Respeaker Zero Case (Autodesk Fusion 360 design; units mm, degrees)
Autodesk Fusion 360 part; units mm, degrees
sketch "Base Bottom" plane through (0, 0, 0) normal (0, 1, 0) x (1, 0, 0)
  line L0 (0, 0) -> (66.3, 0)
  line L1 (66.3, 0) -> (66.3, -31)
  line L2 (66.3, -31) -> (0, -31)
  line L3 (0, -31) -> (0, 0)
  line L4 (-2, -33) -> (68.3, -33)
  line L5 (68.3, -33) -> (68.3, 2)
  line L6 (68.3, 2) -> (-2, 2)
  line L7 (-2, 2) -> (-2, -33)
  line L8 (60, -31) -> (50, -31)
  line L9 (50, -31) -> (50, -33)
  line L10 (50, -33) -> (60, -33)
  line L11 (60, -33) -> (60, -31)
  line L12 (7.15, -7.5) -> (59.15, -7.5)
  line L13 (59.15, -7.5) -> (59.15, 0)
  line L14 (59.15, 0) -> (7.15, 0)
  line L15 (7.15, 0) -> (7.15, -7.5)
  line L16 (-2, -20.5) -> (0, -20.5)
  line L17 (0, -20.5) -> (0, -6.5)
  line L18 (0, -6.5) -> (-2, -6.5)
  line L19 (-2, -6.5) -> (-2, -20.5)
  dimension "d1" = 31
  dimension "d2" = 66.3
  dimension "d3" = 2
  dimension "d4" = 2
  dimension "d5" = 2
  dimension "d6" = 2
  dimension "d9" = 10
  dimension "d12" = 52
  dimension "d13" = 7.5
  dimension "d14" = 7.15
  dimension "d38" = 14
  dimension "d39" = 10.5
  dimension "d40" = 50
  constraint horizontal L0
  constraint vertical L1
  constraint horizontal L2
  constraint vertical L3
  constraint coincident L0.start L3.end
  constraint horizontal L4
  constraint vertical L5
  constraint horizontal L6
  constraint vertical L7
  constraint horizontal L8
  constraint vertical L9
  constraint horizontal L10
  constraint vertical L11
  constraint coincident L4 L9.end
  constraint coincident L2 L8.start
  constraint horizontal L12
  constraint vertical L13
  constraint horizontal L14
  constraint vertical L15
  constraint horizontal L16
  constraint vertical L17
  constraint horizontal L18
  constraint vertical L19
  constraint collinear L3 L17
  constraint collinear L7 L19
  constraint collinear L0 L14
  measures "d1" distance of L0.start L2.end
  measures "d2" distance of L0.start L0.end
  measures "d3" distance of L2 L4
  measures "d4" distance of L1 L5
  measures "d5" distance of L0 L6
  measures "d6" distance of L3 L7
  measures "d9" distance of L8.start L8.end
  measures "d12" distance of L12.start L12.end
  measures "d13" distance of L12.start L14.end
  measures "d14" horizontal distance of L0.start L14.end
  measures "d38" distance of L16.start L18.end
  measures "d39" distance of L2.end L16.end
  measures "d40" distance of L2.end L8.end
  measures "d53" distance of L0.end
  measures "d63" distance of L0.end
  measures "d64" distance of L0.end
extrude "Extrude1" add sketch "Base Bottom" along normal blind 1 makes body 1
extrude "Extrude2" add sketch "Base Bottom" along normal blind 3.5 contours L0 L1 L2 L3 L8 L12 L13 L15 L17 bodies 1
extrude "Extrude3" add sketch "Base Bottom" along normal blind 14 contours L0 L1 L2 L3 L4 L5 L6 L7 L11 L14 L18 | L3 L7 L16 L17 L18 L19 | L2 L3 L4 L7 L9 L16 | L2 L4 L8 L9 L10 L11 bodies 1
sketch "Base Back USB" plane through (0, 0, 33) normal (0, 0, 1) x (-1, 0, 0)
  line L0 (2, 0) -> (-68.3, 0)
  line L1 (-68.3, 0) -> (-68.3, -14)
  line L2 (-68.3, -14) -> (2, -14)
  line L3 (2, -14) -> (2, 0)
  line L4 (-50, -3.5) -> (-60, -3.5)
  line L5 (-60, -3.5) -> (-60, -9.5)
  line L6 (-60, -9.5) -> (-50, -9.5)
  line L7 (-50, -9.5) -> (-50, -3.5)
  line L8 (2, 0) -> (-68.3, 0)
  dimension "d22" = 10
  dimension "d23" = 6
  dimension "d27" = 3.5
  dimension "d41" = 52
  constraint horizontal L4
  constraint vertical L5
  constraint horizontal L6
  constraint vertical L7
  measures "d22" distance of L4.start L4.end
  measures "d23" distance of L4.start L6.end
  measures "d27" distance of L4.start L8
  measures "d41" distance of L3 L6.end
ref_plane "WorkPlane1" through (33.15, 3.5, 15.5) normal (0, 1, 0) x (0, 0, 1)
extrude "Extrude4" cut sketch "Base Back USB" against normal blind 13 contours L4 L5 L6 L7 bodies 1
sketch "Base Side SD" plane through (-2, 0, 0) normal (-1, 0, 0) x (0, -1, 0)
  line L0 (0, -2) -> (0, 33)
  line L1 (0, 33) -> (-14, 33)
  line L2 (-14, 33) -> (-14, -2)
  line L3 (-14, -2) -> (0, -2)
  line L4 (-8, 20.5) -> (-4, 20.5)
  line L5 (-4, 20.5) -> (-4, 6.5)
  line L6 (-4, 6.5) -> (-8, 6.5)
  line L7 (-8, 6.5) -> (-8, 20.5)
  line L8 (0, 6.5) -> (0, 20.5)
  point P0 (0, 33)
  dimension "d42" = 14
  dimension "d43" = 4
  dimension "d44" = 4
  dimension "d127" = 8.5
  constraint horizontal L4
  constraint vertical L5
  constraint horizontal L6
  constraint vertical L7
  measures "d42" distance of L4.start L6.end
  measures "d43" distance of L4.start L4.end
  measures "d44" distance of L5 L8
  measures "d127" distance of L3 L6
extrude "Extrude6" cut sketch "Base Side SD" against normal blind 4 contours L4 L5 L6 L7 bodies 1
sketch "Base Front Mic" plane through (0, 0, -2) normal (0, 0, -1) x (1, 0, 0)
  line L0 (68.3, 0) -> (-2, 0)
  line L1 (-2, 0) -> (-2, -14)
  line L2 (-2, -14) -> (68.3, -14)
  line L3 (68.3, -14) -> (68.3, 0)
  line L4 (64.8, -10.35) -> (59.8, -10.35)
  line L5 (59.8, -10.35) -> (59.8, -14)
  line L6 (59.8, -14) -> (64.8, -14)
  line L7 (64.8, -14) -> (64.8, -10.35)
  line L8 (68.3, 0) -> (-2, 0)
  line L9 (1.5, -10.35) -> (6.5, -10.35)
  line L10 (6.5, -10.35) -> (6.5, -14)
  line L11 (6.5, -14) -> (1.5, -14)
  line L12 (1.5, -14) -> (1.5, -10.35)
  dimension "d48" = 3.5
  dimension "d49" = 10.35
  dimension "d50" = 5
  dimension "d51" = 3.5
  dimension "d52" = 10.35
  dimension "d53" = 5
  constraint horizontal L4
  constraint vertical L5
  constraint horizontal L6
  constraint vertical L7
  constraint coincident L2 L6.end
  constraint horizontal L9
  constraint vertical L10
  constraint horizontal L11
  constraint vertical L12
  constraint coincident L2 L11.end
  measures "d48" distance of L3 L7
  measures "d49" distance of L4 L8
  measures "d50" distance of L4.start L4.end
  measures "d51" distance of L1 L12
  measures "d52" distance of L8 L9
  measures "d53" distance of L10.end L11.end
extrude "Extrude7" cut sketch "Base Front Mic" against normal blind 4 contours L2 L4 L5 L6 L7 | L2 L9 L10 L11 L12 bodies 1
sketch "Base Side Serial" plane through (68.3, 0, 0) normal (1, 0, 0) x (0, 1, 0)
  line L0 (0, 33) -> (0, -2)
  line L1 (0, -2) -> (14, -2)
  line L2 (14, -2) -> (14, 33)
  line L3 (14, 33) -> (0, 33)
  line L4 (4, 24.5) -> (8, 24.5)
  line L5 (8, 24.5) -> (8, 6.5)
  line L6 (8, 6.5) -> (4, 6.5)
  line L7 (4, 6.5) -> (4, 24.5)
  dimension "d113" = 4
  dimension "d114" = 18
  dimension "d115" = 4
  dimension "d128" = 8.5
  constraint horizontal L4
  constraint vertical L5
  constraint horizontal L6
  constraint vertical L7
  measures "d113" distance of L4.start L4.end
  measures "d114" distance of L4.end L5.end
  measures "d115" distance of L0 L7
  measures "d128" distance of L1 L6
extrude "Extrude14" cut sketch "Base Side Serial" against normal blind 10 contours L4 L5 L6 L7 bodies 1
sketch "Cap" plane through (0, 0, 0) normal (0, 1, 0) x (1, 0, 0)
  line L0 (0, 0) -> (66.3, 0)
  line L1 (66.3, 0) -> (66.3, -31)
  line L2 (66.3, -31) -> (0, -31)
  line L3 (0, -31) -> (0, 0)
  line L4 (68.3, -33) -> (-2, -33)
  line L5 (-2, -33) -> (-2, 2)
  line L6 (-2, 2) -> (68.3, 2)
  line L7 (68.3, 2) -> (68.3, -33)
  line L8 (64.3, -29) -> (2, -29)
  line L9 (2, -29) -> (2, -2)
  line L10 (2, -2) -> (64.3, -2)
  line L11 (64.3, -2) -> (64.3, -29)
  line L12 (64.8, -10.5) -> (61.3, -10.5)
  line L13 (61.3, -10.5) -> (61.3, 0)
  line L14 (61.3, 0) -> (64.8, 0)
  line L15 (64.8, 0) -> (64.8, -10.5)
  line L16 (64.8, -10.5) -> (60.3, -10.5)
  line L17 (60.3, -10.5) -> (60.3, -11.5)
  line L18 (60.3, -11.5) -> (64.8, -11.5)
  line L19 (64.8, -11.5) -> (64.8, -10.5)
  line L20 (5, -10.5) -> (1.5, -10.5)
  line L21 (1.5, -10.5) -> (1.5, 0)
  line L22 (1.5, 0) -> (5, 0)
  line L23 (5, 0) -> (5, -10.5)
  line L24 (1.5, -10.5) -> (6, -10.5)
  line L25 (6, -10.5) -> (6, -11.5)
  line L26 (6, -11.5) -> (1.5, -11.5)
  line L27 (1.5, -11.5) -> (1.5, -10.5)
  line L28 (6, -10.5) -> (5, -10.5)
  line L29 (5, -10.5) -> (5, 0)
  line L30 (5, 0) -> (6.5, 0)
  line L31 (64.8, -10.5) -> (66.3, -10.5)
  line L32 (66.3, -10.5) -> (66.3, -11.5)
  line L33 (66.3, -11.5) -> (64.8, -11.5)
  line L34 (64.8, -11.5) -> (64.8, -10.5)
  line L35 (1.5, -11.5) -> (0, -11.5)
  line L36 (0, -11.5) -> (0, -10.5)
  line L37 (0, -10.5) -> (1.5, -10.5)
  line L38 (1.5, -10.5) -> (1.5, -11.5)
  circle A0 centre (49, -12.4) radius 3.3
  line L39 (66.3, -11.5) -> (64.3, -11.5)
  line L40 (64.3, -11.5) -> (64.3, -21)
  line L41 (64.3, -21) -> (66.3, -21)
  line L42 (66.3, -21) -> (66.3, -11.5)
  line L43 (1.5, 0) -> (6.5, 0)
  line L44 (6.5, 0) -> (6.5, 2)
  line L45 (6.5, 2) -> (1.5, 2)
  line L46 (1.5, 2) -> (1.5, 0)
  line L47 (59.8, 0) -> (64.8, 0)
  line L48 (64.8, 0) -> (64.8, 2)
  line L49 (64.8, 2) -> (59.8, 2)
  line L50 (59.8, 2) -> (59.8, 0)
  line L51 (5, -10.5) -> (6, -10.5)
  line L52 (6, -10.5) -> (6, -7.3)
  line L53 (6, -7.3) -> (5, -7.3)
  line L54 (5, -7.3) -> (5, -10.5)
  line L55 (5, -7.3) -> (6.5199, 0.1987)
  line L56 (6.5199, 0.1987) -> (7.5, 0)
  line L57 (7.5, 0) -> (5.9801, -7.4987)
  line L58 (5.9801, -7.4987) -> (5, -7.3)
  line L59 (61.3, -10.5) -> (60.3, -10.5)
  line L60 (60.3, -10.5) -> (60.3, -7.3)
  line L61 (60.3, -7.3) -> (61.3, -7.3)
  line L62 (61.3, -7.3) -> (61.3, -10.5)
  line L63 (61.3, -7.3) -> (59.7801, 0.1987)
  line L64 (59.7801, 0.1987) -> (58.8, 0)
  line L65 (58.8, 0) -> (60.3199, -7.4987)
  line L66 (60.3199, -7.4987) -> (61.3, -7.3)
  dimension "d56" = 66.3
  dimension "d57" = 31
  dimension "d58" = 2
  dimension "d59" = 2
  dimension "d60" = 2
  dimension "d61" = 2
  dimension "d62" = 2
  dimension "d63" = 2
  dimension "d64" = 2
  dimension "d65" = 2
  dimension "d72" = 3.5
  dimension "d73" = 3.5
  dimension "d74" = 10.5
  dimension "d75" = 4.5
  dimension "d76" = 1
  dimension "d78" = 3.5
  dimension "d79" = 3.5
  dimension "d80" = 10.5
  dimension "d81" = 4.5
  dimension "d82" = 1
  dimension "d103" = 6.6
  dimension "d105" = 14.4
  dimension "d108" = 19.3
  dimension "d109" = 9.5
  dimension "d129" = 3.5
  dimension "d130" = 5
  dimension "d131" = 5
  dimension "d132" = 3.5
  dimension "d137" = 1
  dimension "d138" = 3.2
  dimension "d139" = 1
  dimension "d140" = 6
  dimension "d141" = 1
  dimension "d142" = 3.2
  dimension "d143" = 1
  dimension "d144" = 6
  constraint horizontal L0
  constraint vertical L1
  constraint horizontal L2
  constraint vertical L3
  constraint coincident L0.start L3.end
  constraint horizontal L4
  constraint vertical L5
  constraint horizontal L6
  constraint vertical L7
  constraint horizontal L8
  constraint vertical L9
  constraint horizontal L10
  constraint vertical L11
  constraint horizontal L12
  constraint vertical L13
  constraint horizontal L14
  constraint vertical L15
  constraint coincident L0 L13.end
  constraint horizontal L16
  constraint vertical L17
  constraint horizontal L18
  constraint vertical L19
  constraint horizontal L20
  constraint vertical L21
  constraint horizontal L22
  constraint vertical L23
  constraint coincident L0 L21.end
  constraint horizontal L24
  constraint vertical L25
  constraint horizontal L26
  constraint vertical L27
  constraint horizontal L28
  constraint vertical L29
  constraint horizontal L30
  constraint horizontal L31
  constraint vertical L32
  constraint horizontal L33
  constraint vertical L34
  constraint coincident L1 L32.end
  constraint horizontal L35
  constraint vertical L36
  constraint horizontal L37
  constraint vertical L38
  constraint coincident L3 L36.end
  constraint horizontal L39
  constraint vertical L40
  constraint horizontal L41
  constraint vertical L42
  constraint collinear L11 L40
  constraint horizontal L43
  constraint vertical L44
  constraint horizontal L45
  constraint vertical L46
  constraint collinear L0 L43
  constraint collinear L6 L45
  constraint horizontal L47
  constraint vertical L48
  constraint horizontal L49
  constraint vertical L50
  constraint collinear L0 L47
  constraint collinear L6 L49
  constraint horizontal L51
  constraint vertical L52
  constraint horizontal L53
  constraint vertical L54
  constraint perpendicular L55 L56
  constraint parallel L55 L57
  constraint parallel L56 L58
  constraint coincident L0 L56.end
  constraint horizontal L59
  constraint vertical L60
  constraint horizontal L61
  constraint vertical L62
  constraint perpendicular L63 L64
  constraint parallel L63 L65
  constraint parallel L64 L66
  constraint coincident L0 L64.end
  measures "d56" distance of L1.end L2.end
  measures "d57" distance of L0.end L1.end
  measures "d58" distance of L2 L4
  measures "d59" distance of L3 L5
  measures "d60" distance of L0 L6
  measures "d61" distance of L1 L7
  measures "d62" distance of L2 L8
  measures "d63" distance of L1 L11
  measures "d64" distance of L0 L10
  measures "d65" distance of L3 L9
  measures "d72" distance of L7 L15
  measures "d73" distance of L12.start L12.end
  measures "d74" distance of L12.end L13.end
  measures "d75" distance of L12.start L16.end
  measures "d76" distance of L12.start L18.end
  measures "d78" distance of L5 L21
  measures "d79" distance of L20.start L20.end
  measures "d80" distance of L20.start L22.end
  measures "d81" distance of L20.end L24.end
  measures "d82" distance of L20.end L26.end
  measures "d103" diameter of A0
  measures "d105" distance of L6 A0.centre
  measures "d108" distance of L7 A0.centre
  measures "d109" distance of L32.end L41.end
  measures "d129" distance of L5 L46
  measures "d130" distance of L44.end L45.end
  measures "d131" distance of L48.end L49.end
  measures "d132" distance of L7 L48
  measures "d137" distance of L20.start L24.end
  measures "d138" distance of L20.start L53.end
  measures "d139" distance of L53.end L57.end
  measures "d140" distance of L21 L56.end
  measures "d141" distance of L12.end L16.end
  measures "d142" distance of L16.end L60.end
  measures "d143" distance of L61.end L65.end
  measures "d144" distance of L15 L64.end
extrude "Extrude8" add sketch "Cap" along normal blind 2 separate body contours L0 L1 L2 L3 L4 L5 L6 L7 L32 L36 L42 L46 L48 | L0 L3 L21 L37 | L0 L6 L22 L30 L43 L44 L45 L46 L55 | L0 L9 L10 L20 L21 L22 L23 L24 L29 L43 | L3 L27 L35 L36 L37 L38 | L0 L10 L23 L29 L30 L43 L55 | L9 L20 L24 L26 L27 L38 | L1 L2 L3 L8 L9 L11 L26 L35 L41 | L0 L30 L43 L44 L55 | L0 L10 L30 L43 L55 L57 | L9 L10 L20 L23 L24 L29 L54 | L10 L23 L29 L55 | L9 L20 L24 L25 L26 L28 L51 | L0 L6 L44 L50 L55 L56 L63 L64 | L0 L44 L55 L56 | L10 L52 L53 L55 L57 | L23 L24 L28 L29 L51 L52 L54 L57 L58 | L52 L53 L57 L58 | L8 L9 L10 L11 L17 L18 L25 L26 L40 L52 L57 L60 L65 | L0 L6 L14 L47 L48 L49 L50 L63 | L0 L10 L57 L65 | L0 L47 L50 L63 | L0 L50 L63 L64 | L1 L11 L18 L33 L39 L40 L41 L42 | L0 L10 L47 L63 L65 | L10 L60 L61 L63 L65 | L0 L10 L11 L12 L13 L14 L15 L16 L47 | L0 L1 L15 L31 | L0 L10 L13 L47 L63 | L1 L19 L31 L32 L33 L34 L39 | L10 L13 L63 | L13 L16 L59 L60 L62 L65 L66 | L60 L61 L65 L66 | L11 L12 L16 L18 L19 L34 L39 | L11 L12 L16 L17 L18 L59 | L10 L11 L12 L13 L16 L62 | A0 makes body 2
extrude "Extrude9" add sketch "Cap" along normal blind 4 contours L0 L3 L21 L37 | L0 L9 L10 L20 L21 L22 L23 L24 L29 L43 | L3 L27 L35 L36 L37 L38 | L0 L10 L23 L29 L30 L43 L55 | L9 L20 L24 L26 L27 L38 | L1 L2 L3 L8 L9 L11 L26 L35 L41 | L0 L10 L30 L43 L55 L57 | L0 L10 L57 L65 | L1 L11 L18 L33 L39 L40 L41 L42 | L0 L10 L47 L63 L65 | L0 L10 L11 L12 L13 L14 L15 L16 L47 | L0 L1 L15 L31 | L0 L10 L13 L47 L63 | L1 L19 L31 L32 L33 L34 L39 | L11 L12 L16 L18 L19 L34 L39 bodies 2
extrude "Extrude10" cut sketch "Cap" along normal blind 2 from surface at 2 contours L0 L9 L10 L20 L21 L22 L23 L24 L29 L43 | L0 L10 L23 L29 L30 L43 L55 | L0 L10 L47 L63 L65 | L0 L10 L11 L12 L13 L14 L15 L16 L47 | L0 L10 L13 L47 L63 bodies 2
extrude "Extrude11" add sketch "Cap" along normal blind 3.6 from surface at 2 contours L0 L3 L21 L37 | L3 L27 L35 L36 L37 L38 | L9 L20 L24 L26 L27 L38 | L0 L10 L30 L43 L55 L57 | L9 L20 L24 L25 L26 L28 L51 | L10 L52 L53 L55 L57 | L23 L24 L28 L29 L51 L52 L54 L57 L58 | L52 L53 L57 L58 | L0 L10 L47 L63 L65 | L10 L60 L61 L63 L65 | L0 L1 L15 L31 | L1 L19 L31 L32 L33 L34 L39 | L13 L16 L59 L60 L62 L65 L66 | L60 L61 L65 L66 | L11 L12 L16 L18 L19 L34 L39 | L11 L12 L16 L17 L18 L59 bodies 2
extrude "Extrude12" cut sketch "Cap" along normal blind 6 contours A0 bodies 2
extrude "Extrude13" cut sketch "Cap" along normal blind 3 from surface at 2 contours L1 L11 L18 L33 L39 L40 L41 L42 bodies 2
fillet "Fillet1" radius 4.5 2 edges at (63.05, 2, 10.5) (3.25, 2, 10.5) on bodies 2
copy_body "Body->Comp1" bodies 1 removing the originals makes body 3 in component "Base"
copy_body "Body->Comp2" bodies 2 removing the originals makes body 4 in component "Cap"
chamfer "Chamfer1" distance 2 angle 45 6 edges at (62.3, 10.35, -2) (64.8, 12.175, -2) (59.8, 12.175, -2) (6.5, 12.175, -2) (4, 10.35, -2) (1.5, 12.175, -2) on bodies 3 in component "Base"
fillet "Fillet2" radius 2 4 edges at (-2, 7, -2) (-2, 7, 33) (68.3, 7, 33) (68.3, 7, -2) on bodies 3 in component "Base"
fillet "Fillet1'" radius 2 4 edges at (-2, 1, -2) (68.3, 1, -2) (68.3, 1, 33) (-2, 1, 33) on bodies 4 in component "Cap"
fillet "Fillet4" radius 1.5 12 edges at (67.3, 8, 24.5) (-1, 8, 20.5) (-1, 4, 20.5) (-1, 8, 6.5) (-1, 4, 6.5) (67.3, 4, 24.5) (50, 9.5, 32) (67.3, 8, 6.5) (50, 3.5, 32) (67.3, 4, 6.5) (60, 3.5, 32) (60, 9.5, 32) on bodies 3 in component "Base"
component "Base" placed x (1, 0, 0) y (0, 1, 0) z (0, 0, 1) at (0, 0, 0)
component "Cap" placed x (-1, 0, 0) y (0, -1, 0) z (0, 0, 1) at (66.3, 16, 0)
named bodies: "Base", "Cap"
